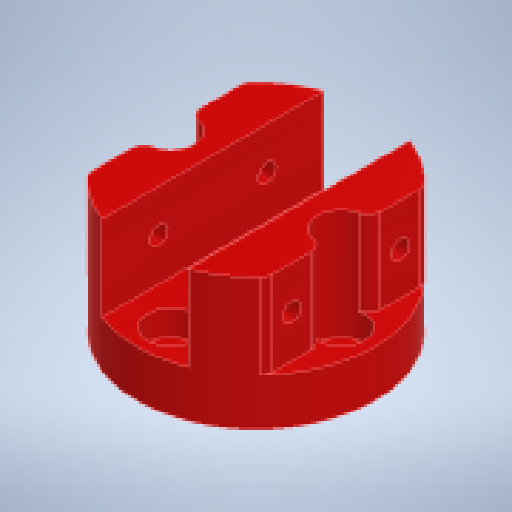
# Autodesk Inventor part: Acople Antena - Motor
Saved by Autodesk Inventor 2023 (Build 270158000, 158)
## iProperties
Created: 2023-11-07
Part Number: Acople Antena - Motor
Material: PET Plastic
Document SubType Name: Modeling
Designer: juanp
Density: 1.541 g/cm^3
Appearance: Red
Author: juanp
Autodesk Inventor part; units mm, degrees
ref_plane "YZ Plane" through (0, 0, 0) normal (1, 0, 0) x (0, 1, 0)
ref_plane "XZ Plane" through (0, 0, 0) normal (0, 1, 0) x (-1, 0, 0)
ref_plane "XY Plane" through (0, 0, 0) normal (0, 0, 1) x (1, 0, 0)
sketch "Sketch1" plane through (0, 0, 0) normal (0, 1, 0) x (-1, 0, 0)
  line L0 (28, 28) -> (-28, 28) construction
  line L1 (-28, 28) -> (-28, -28) construction
  line L2 (-28, -28) -> (28, -28) construction
  line L3 (28, -28) -> (28, 28) construction
  line L4 (28, 28) -> (-28, -28) construction
  line L5 (-28, 28) -> (28, -28) construction
  circle A0 centre (0, 0) radius 28
  circle A1 centre (0, 0) radius 15 construction
  circle A2 centre (0, 0) radius 8.5
  line L6 (0, 0) -> (0, 20) construction
  circle A3 centre (0, 20) radius 2.5
  circle A4 centre (0, 0) radius 4.15
  line L7 (0, 0) -> (-14.1421, 14.1421) construction
  circle A5 centre (-14.1421, 14.1421) radius 2.5
  line L8 (0, 0) -> (-20, 0) construction
  circle A6 centre (-20, 0) radius 2.5
  line L9 (0, 0) -> (-14.1421, -14.1421) construction
  circle A7 centre (-14.1421, -14.1421) radius 2.5
  line L10 (0, 0) -> (0, -20) construction
  circle A8 centre (0, -20) radius 2.5
  line L11 (0, 0) -> (14.1421, -14.1421) construction
  circle A9 centre (14.1421, -14.1421) radius 2.5
  line L12 (0, 0) -> (20, 0) construction
  circle A10 centre (20, 0) radius 2.5
  line L13 (0, 0) -> (14.1421, 14.1421) construction
  circle A11 centre (14.1421, 14.1421) radius 2.5
  circle A12 centre (0, 20) radius 5.5
  circle A13 centre (-14.1421, 14.1421) radius 5.5
  circle A14 centre (-20, 0) radius 5.5
  circle A15 centre (-14.1421, -14.1421) radius 5.5
  circle A16 centre (0, -20) radius 5.5
  circle A17 centre (14.1421, -14.1421) radius 5.5
  circle A18 centre (20, 0) radius 5.5
  circle A19 centre (14.1421, 14.1421) radius 5.5
  line L14 (10.15, 28) -> (-10.15, 28) construction
  line L15 (-10.15, 28) -> (-10.15, -28)
  line L16 (-10.15, -28) -> (10.15, -28) construction
  line L17 (10.15, -28) -> (10.15, 28)
  line L18 (10.15, 28) -> (-10.15, -28) construction
  line L19 (-10.15, 28) -> (10.15, -28) construction
  line L20 (-21.15, 28) -> (21.15, 28) construction
  line L21 (21.15, 28) -> (21.15, -28)
  line L22 (21.15, -28) -> (-21.15, -28) construction
  line L23 (-21.15, -28) -> (-21.15, 28)
  line L24 (-21.15, 28) -> (21.15, -28) construction
  line L25 (21.15, 28) -> (-21.15, -28) construction
  point P0 (0, 0)
  point P1 (0, 0)
  point P2 (-28, 0)
  point P3 (0, 28)
  point P4 (28, 0)
  point P5 (0, -28)
  point P6 (0, 28)
  point P7 (0, -28)
  point P8 (25.7633, 10.966)
  point P9 (25.7633, -10.966)
  point P10 (-25.7633, -10.966)
  point P11 (-25.7633, 10.966)
  point P12 (0, 0)
  point P13 (-10.15, -26.0955)
  point P14 (-10.15, 26.0955)
  point P15 (10.15, 26.0955)
  point P16 (10.15, -26.0955)
  point P17 (21.15, -18.3488)
  point P18 (21.15, -5.3784)
  point P19 (21.15, 5.3784)
  point P20 (21.15, 18.3488)
  point P21 (-21.15, 18.3488)
  point P22 (-21.15, 5.3784)
  point P23 (-21.15, -5.3784)
  point P24 (-21.15, -18.3488)
  dimension "d4" = 56
  dimension "d5" = 30
  dimension "d6" = 17
  dimension "d7" = 20
  dimension "d8" = 5
  dimension "d9" = 8.3
  dimension "d10" = 360
  dimension "d51" = 3
  dimension "d54" = 360
  dimension "d66" = 20.3
  dimension "d67" = 11
  dimension "d71" = 11
  constraints: 52 end point, 20 centre point, 15 coincident, 10 midpoint, 6 parallel, 4 point on circle, 3 horizontal, 3 perpendicular, 3 tangent, 1 collinear, 1 vertical, 56 other
  measures "d4" diameter of A0
  measures "d5" diameter of A1
  measures "d6" diameter of A2
  measures "d7" distance of L6.start L6.end
  measures "d8" diameter of A3
  measures "d9" diameter of A4
  measures "d51" radial gap between concentric circles of A3 A12
  measures "d66" distance between parallel lines of L17 L15
  measures "d67" distance between parallel lines of L17 L21
  measures "d71" diameter of A12
extrude "Extrusion1" add sketch "Sketch1" against normal blind 5 contours A0 L21 A18 | L21 A18 A0 L17 A17 A19 | L17 A19 A17 A0 L15 A15 A13 | L21 A10 A18 | A18 L21 A10 | L15 A13 A15 A0 L23 A14 | L17 A19 | A19 L17 | L17 A17 | A17 L17 | L23 A14 A0 | L15 A13 | A13 L15 | L15 A15 | A15 L15 | L23 A6 A14 | A14 L23 A6 | A2 | A5 | A7 | A9 | A11 | A12 | A16
extrude "Extrusion8" add sketch "Sketch1" along normal blind 26 contours L21 A18 A0 L17 A17 A19 | L15 A13 A15 A0 L23 A14 | A19 L17 | L17 A17 | L15 A13 | A15 L15 | A5 | A7 | A9 | A11 picked at (10.6474, 14.1421) picked at (10.6474, -14.1421) picked at (-10.6474, 14.1421) picked at (-10.6474, -14.1421)
extrude "Extrusion9" add sketch "Sketch1" along normal blind 6 contours A0 L21 A18 | L17 A19 A17 A0 L15 A15 A13 | L17 A19 | A17 L17 | L23 A14 A0 | A13 L15 | L15 A15 | A2 picked at (9.6581, 14.3404) picked at (9.91, -15.0875) picked at (-9.4335, 13.8687) picked at (-9.6474, -14.1421)
fillet "Fillet2" radius 3 8 edges at (-21.15, 16, 5.3784) (-21.15, 16, -5.3784) (21.15, 16, 5.3784) (21.15, 16, -5.3784) (21.15, 16, 18.3488) (21.15, 16, -18.3488) (-21.15, 16, 18.3488) (-21.15, 16, -18.3488)
sketch "Sketch9" plane through (-21.15, 6, -17.1924) normal (-1, 0, 0) x (0, 0, 1)
  line L0 (0, 20) -> (0, 0) projected
  line L1 (8.8961, 20) -> (8.8961, 0) projected
  line L2 (0, 20) -> (8.8961, 0) construction
  line L3 (25.4886, 20) -> (25.4886, 0) projected
  line L4 (34.3847, 0) -> (34.3847, 20) projected
  line L5 (25.4886, 20) -> (34.3847, 0) construction
  circle A0 centre (4.4481, 10) radius 2.15
  circle A1 centre (29.9367, 10) radius 2.15
  point P0 (17.1924, -6)
  dimension "d72" = 4.3
  constraints: 4 end point, 2 centre point, 2 midpoint, 1 equal radius
  measures "d72" diameter of A0
extrude "Extrusion10" cut sketch "Sketch9" against normal through all
body "Solid1"
